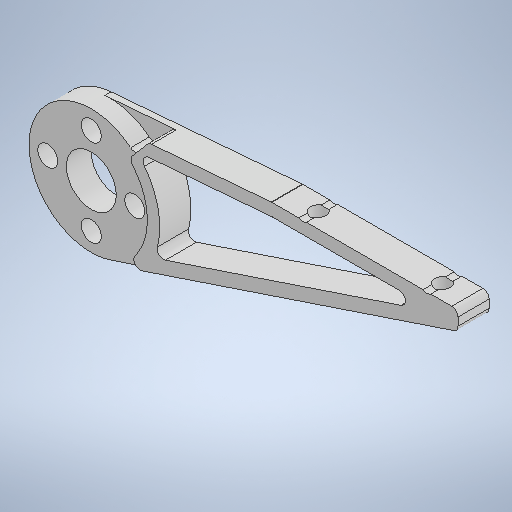
# Autodesk Inventor part: T5.0_club-face
Saved by Autodesk Inventor 2025 (Build 290162000, 162)
## iProperties
Created: 2024-07-26
Part Number: T5.0_club-face
Material: 一般
Document SubType Name: Sheet Metal
Designer: 8326d
Density: 1 g/cm^3
Sheet Metal Rule: Default_mm
Appearance: 既定
Author: 8326d
Autodesk Inventor part; units mm, degrees
ref_plane "YZ Plane" through (0, 0, 0) normal (1, 0, 0) x (0, 1, 0)
ref_plane "XZ Plane" through (0, 0, 0) normal (0, 1, 0) x (-1, 0, 0)
ref_plane "XY Plane" through (0, 0, 0) normal (0, 0, 1) x (1, 0, 0)
sketch "スケッチ1" plane through (0, 0, 0) normal (0, 0, 1) x (1, 0, 0)
  circle A0 centre (0, 0) radius 10
  line L0 (30, 12.5) -> (60, 12.5)
  line L1 (60, 12.5) -> (60, 9.5)
  line L2 (60, 9.5) -> (30, 9.5)
  line L3 (30, 9.5) -> (30, 12.5)
  line L4 (30, 12.5) -> (-0.819325, 9.966379)
  line L5 (3.168424, -9.484782) -> (60, 9.5)
  dimension "d0" = 20
  dimension "d1" = 30
  dimension "d2" = 3
  dimension "d3" = 12.5
  dimension "d4" = 60
  measures "d0" diameter of A0
  measures "d1" distance of L1.end L2.end
  measures "d2" distance of L0.end L1.end
  measures "d3" distance from line of L0 point (0, 0)
  measures "d4" distance from line of point (0, 0) L1
extrude "プレート1" add sketch "スケッチ1" along normal blind 5
sketch "スケッチ2" plane through (0, 0, 5) normal (0, 0, 1) x (1, 0, 0)
  arc A0 (-0.819325, 9.966379) -> (3.168424, -9.484782) centre (0, 0) ccw
  line L0 (30, 12.5) -> (-0.819325, 9.966379)
  circle A1 centre (0, 0) radius 10
  point P0 (3.168424, -9.484782)
  constraints: 1 coincident, 3 other
extrude "押し出し1" cut sketch "スケッチ2" against normal blind 1
sketch "スケッチ3" plane through (0, 0, 4) normal (0, 0, 1) x (1, 0, 0)
  circle A0 centre (0, 0) radius 7 construction
  line L0 (0, -7) -> (7, 0) construction
  line L1 (7, 0) -> (0, 7) construction
  line L2 (0, 7) -> (-7, 0) construction
  line L3 (-7, 0) -> (0, -7) construction
  line L4 (0, -7) -> (0, 7) construction
  line L5 (7, 0) -> (-7, 0) construction
  dimension "d8" = 14
  constraints: 12 end point, 5 coincident, 2 midpoint, 2 parallel, 2 perpendicular, 1 vertical, 1 vertical alignment, 2 other
hole "穴1" at (0, 7, 4) at (7, 0, 4) at (0, -7, 4) at (-7, 0, 4) direction (0, 0, -1) diameter 3.2 end through all
sketch "スケッチ4" plane through (0, 0, 4) normal (0, 0, 1) x (1, 0, 0)
  circle A0 centre (0, 0) radius 4
  dimension "d16" = 8
  constraints: 1 centre point, 1 coincident
  measures "d16" diameter of A0
extrude "押し出し2" cut sketch "スケッチ4" against normal through all
sketch "スケッチ6" plane through (0, 0, 5) normal (0, 0, 1) x (1, 0, 0)
  line L0 (60, 9.5) -> (3.168424, -9.484782)
  line L1 (60, 12.5) -> (60, 9.5)
  line L2 (30, 12.5) -> (60, 12.5)
  line L3 (-0.819325, 9.966379) -> (30, 12.5)
  arc A0 (3.168424, -9.484782) -> (-0.819325, 9.966379) centre (0, 0) ccw
  line L4 (30.08207, 10.5) -> (56.681246, 10.5)
  line L5 (56.681246, 10.5) -> (11.018186, -4.753901)
  arc A1 (11.018186, -4.753901) -> (8.258741, 8.705929) centre (0, 0) ccw
  line L6 (8.258741, 8.705929) -> (30.08207, 10.5)
  dimension "d28" = 2
  constraints: 6 end point, 2 point on circle, 1 centre point, 3 other
  measures "d28" distance between parallel lines of L3 L6
extrude "押し出し4" cut sketch "スケッチ6" against normal through all contours L4 L5 A1 L6
sketch "スケッチ5" plane through (0, 0, 5) normal (0, 0, 1) x (1, 0, 0)
  line L0 (30, 12.5) -> (60, 12.5) projected
  circle A0 centre (35, 13.35) radius 1.05
  circle A1 centre (55, 13.35) radius 1.05
  line L1 (60, 12.5) -> (60, 9.5) projected
  point P0 (0, 0)
  dimension "d20" = 2.1
  dimension "d21" = 2.1
  dimension "d22" = 5
  dimension "d23" = 5
  dimension "d24" = 0.85
  dimension "d25" = 0.85
  constraints: 2 centre point
  measures "d20" diameter of A0
  measures "d21" diameter of A1
  measures "d22" horizontal distance of L0.start A0.centre
  measures "d23" distance from line of L1 A1.centre
  measures "d24" distance from line of L0 A0.centre
  measures "d25" distance from line of L0 A1.centre
extrude "押し出し3" cut sketch "スケッチ5" against normal through all
fillet "フィレット2" radius 1 4 edges at (11.0182, -4.7539, 2.5) (8.2587, 8.7059, 2.5) (56.6812, 10.5, 2.5) (30.0821, 10.5, 2.5)
sketch "スケッチ7" plane through (35.616441, 12.5, 0) normal (0, 1, 0) x (1, 0, 0)
  line L0 (18.767117, -5) -> (18.767117, 0)
  line L1 (20, -5) -> (18.767117, -5)
  line L2 (20, 0) -> (20, -5)
  line L3 (18.767117, 0) -> (20, 0)
  line L4 (-1.232883, -5) -> (-1.232883, 0)
  line L5 (0, -5) -> (-1.232883, -5)
  line L6 (0, 0) -> (0, -5)
  line L7 (-1.232883, 0) -> (0, 0)
  point P0 (-35.616441, 0)
  point P1 (-0.616441, -2.5)
  point P2 (19.383559, -2.5)
  point P3 (19.383559, -5)
  point P4 (-0.616441, -5)
  point P5 (-1.232883, -2.5)
  point P6 (18.767117, -2.5)
  constraints: 4 midpoint, 2 horizontal alignment, 2 vertical alignment
hole "穴2" at (35, 12.5, 2.5) at (55, 12.5, 2.5) direction (0, -1, 0) diameter 2.5 depth 8 tip angle 118
fillet "フィレット3" radius 1 3 edges at (60, 9.5, 2.5) (60, 12.5, 2.5) (30, 12.5, 2.5)
sketch "スケッチ8" plane through (0, 0, 5) normal (0, 0, 1) x (1, 0, 0)
  arc A0 (3.168424, -9.484782) -> (-0.819325, 9.966379) centre (0, 0) ccw
  line L0 (-0.819325, 9.966379) -> (29.959103, 12.496638)
  line L1 (10.269293, 10.877961) -> (7.054657, 7.08744)
  arc A1 (10.262161, 8.870628) -> (9.548394, 7.268299) centre (10.344094, 7.87399) ccw
  dimension "d40" = 2
  dimension "d41" = 45
  constraints: 2 end point, 1 point on circle, 1 point on line
  measures "d40" distance from line of L1 A1.centre
  measures "d41" angle of L0 L1
extrude "押し出し5" cut sketch "スケッチ8" against normal blind 4
fillet "フィレット4" radius 1 4 edges at (7.0547, 7.0874, 2.5) (7.0547, 7.0874, 4.5) (10.2693, 10.878, 3) (3.1684, -9.4848, 4.5)
equation "\"d14\" = Thickness"
equation "\"d23\" = d22"
equation "\"d25\" = d24"
equation "\"d5\" = Thickness"
equation "\"BendRadius\" = Thickness"
equation "\"BendReliefWidth\" = Thickness"
equation "\"BendReliefDepth\" = 0.5 * Thickness"
equation "\"TransitionRadius\" = BendRadius"
equation "\"JacobiRadiusSize\" = BendRadius"
equation "\"GapSize\" = Thickness"
equation "\"Thickness\" = 5"
